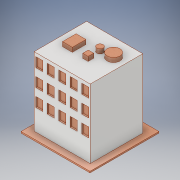
# Autodesk Inventor part: apartment_1
Saved by Autodesk Inventor 2019 (Build 230136000, 136)
## iProperties
Created: 2020-04-29
Part Number: apartment_1
Material: Wood (Oak)
Document SubType Name: Modeling
Designer: infinity
Density: 0.76 g/cm^3
Appearance: White Oak - Natural Medium Gloss
Author: infinity
Autodesk Inventor part; units mm, degrees
ref_plane "YZ Plane" through (0, 0, 0) normal (1, 0, 0) x (0, 1, 0)
ref_plane "XZ Plane" through (0, 0, 0) normal (0, 1, 0) x (-1, 0, 0)
ref_plane "XY Plane" through (0, 0, 0) normal (0, 0, 1) x (1, 0, 0)
sketch "Sketch1" plane through (0, 0, 0) normal (0, 1, 0) x (-1, 0, 0)
  line L0 (0, 0) -> (1219.2, 0)
  line L1 (1219.2, 0) -> (1219.2, -1219.2)
  line L2 (1219.2, -1219.2) -> (0, -1219.2)
  line L3 (0, -1219.2) -> (0, 0)
  dimension "d0" = 1219.2
  dimension "d1" = 1219.2
  constraints: 8 end point, 2 parallel, 1 horizontal, 1 perpendicular
  measures "d0" distance of L0.end L1.end
  measures "d1" distance of L1.end L2.end
extrude "Extrusion1" add sketch "Sketch1" along normal blind 25.4
sketch "Sketch2" plane through (0, 25.4, 0) normal (0, 1, 0) x (1, 0, 0)
  line L0 (-1107.5056, 119.0242) -> (-114.6697, 119.0242)
  line L1 (-114.6697, 119.0242) -> (-114.6697, 1047.9936)
  line L2 (-114.6697, 1047.9936) -> (-1107.5056, 1047.9936)
  line L3 (-1107.5056, 1047.9936) -> (-1107.5056, 119.0242)
  point P0 (0, 0)
  constraints: 8 end point, 2 parallel, 1 horizontal, 1 perpendicular
extrude "Extrusion2" add sketch "Sketch2" along normal blind 1219.2
sketch "Sketch3" plane through (0, 1244.6, 0) normal (0, 1, 0) x (1, 0, 0)
  line L0 (-933.3238, 447.0665) -> (-759.1421, 447.0665)
  line L1 (-759.1421, 447.0665) -> (-759.1421, 688.0179)
  line L2 (-759.1421, 688.0179) -> (-933.3238, 688.0179)
  line L3 (-933.3238, 688.0179) -> (-933.3238, 447.0665)
  line L4 (-576.2513, 447.0665) -> (-480.4513, 447.0665)
  line L5 (-480.4513, 447.0665) -> (-480.4513, 545.7695)
  line L6 (-480.4513, 545.7695) -> (-576.2513, 545.7695)
  line L7 (-576.2513, 545.7695) -> (-576.2513, 447.0665)
  circle A0 centre (-528.3513, 705.4361) radius 55.5572
  circle A1 centre (-317.8817, 734.4664) radius 113.2181
  point P0 (0, 0)
  constraints: 16 end point, 4 parallel, 2 centre point, 2 horizontal, 2 perpendicular, 1 point on line
extrude "Extrusion3" add sketch "Sketch3" along normal blind 76.2
sketch "Sketch4" plane through (-1107.5056, 25.4, -119.0242) normal (0, 0, 1) x (1, 0, 0)
  line L0 (30.4818, 1157.5843) -> (152.4572, 1157.5843)
  line L1 (152.4572, 1157.5843) -> (152.4572, 989.2087)
  line L2 (152.4572, 989.2087) -> (30.4818, 989.2087)
  line L3 (30.4818, 989.2087) -> (30.4818, 1157.5843)
  line L4 (0, 1219.2) -> (992.8359, 1219.2) projected
  line L5 (0, 0) -> (0, 1219.2) projected
  line L6 (233.6818, 1157.5843) -> (355.6572, 1157.5843)
  line L7 (355.6572, 1157.5843) -> (355.6572, 989.2087)
  line L8 (355.6572, 989.2087) -> (233.6818, 989.2087)
  line L9 (233.6818, 989.2087) -> (233.6818, 1157.5843)
  line L10 (436.8818, 1157.5843) -> (558.8572, 1157.5843)
  line L11 (558.8572, 1157.5843) -> (558.8572, 989.2087)
  line L12 (558.8572, 989.2087) -> (436.8818, 989.2087)
  line L13 (436.8818, 989.2087) -> (436.8818, 1157.5843)
  line L14 (640.0818, 1157.5843) -> (762.0572, 1157.5843)
  line L15 (762.0572, 1157.5843) -> (762.0572, 989.2087)
  line L16 (762.0572, 989.2087) -> (640.0818, 989.2087)
  line L17 (640.0818, 989.2087) -> (640.0818, 1157.5843)
  line L18 (843.2818, 1157.5843) -> (965.2572, 1157.5843)
  line L19 (965.2572, 1157.5843) -> (965.2572, 989.2087)
  line L20 (965.2572, 989.2087) -> (843.2818, 989.2087)
  line L21 (843.2818, 989.2087) -> (843.2818, 1157.5843)
  line L22 (30.4818, 852.7843) -> (152.4572, 852.7843)
  line L23 (152.4572, 852.7843) -> (152.4572, 684.4087)
  line L24 (152.4572, 684.4087) -> (30.4818, 684.4087)
  line L25 (30.4818, 684.4087) -> (30.4818, 852.7843)
  line L26 (233.6818, 852.7843) -> (355.6572, 852.7843)
  line L27 (355.6572, 852.7843) -> (355.6572, 684.4087)
  line L28 (355.6572, 684.4087) -> (233.6818, 684.4087)
  line L29 (233.6818, 684.4087) -> (233.6818, 852.7843)
  line L30 (436.8818, 852.7843) -> (558.8572, 852.7843)
  line L31 (558.8572, 852.7843) -> (558.8572, 684.4087)
  line L32 (558.8572, 684.4087) -> (436.8818, 684.4087)
  line L33 (436.8818, 684.4087) -> (436.8818, 852.7843)
  line L34 (640.0818, 852.7843) -> (762.0572, 852.7843)
  line L35 (762.0572, 852.7843) -> (762.0572, 684.4087)
  line L36 (762.0572, 684.4087) -> (640.0818, 684.4087)
  line L37 (640.0818, 684.4087) -> (640.0818, 852.7843)
  line L38 (843.2818, 852.7843) -> (965.2572, 852.7843)
  line L39 (965.2572, 852.7843) -> (965.2572, 684.4087)
  line L40 (965.2572, 684.4087) -> (843.2818, 684.4087)
  line L41 (843.2818, 684.4087) -> (843.2818, 852.7843)
  line L42 (30.4818, 547.9843) -> (152.4572, 547.9843)
  line L43 (152.4572, 547.9843) -> (152.4572, 379.6087)
  line L44 (152.4572, 379.6087) -> (30.4818, 379.6087)
  line L45 (30.4818, 379.6087) -> (30.4818, 547.9843)
  line L46 (233.6818, 547.9843) -> (355.6572, 547.9843)
  line L47 (355.6572, 547.9843) -> (355.6572, 379.6087)
  line L48 (355.6572, 379.6087) -> (233.6818, 379.6087)
  line L49 (233.6818, 379.6087) -> (233.6818, 547.9843)
  line L50 (436.8818, 547.9843) -> (558.8572, 547.9843)
  line L51 (558.8572, 547.9843) -> (558.8572, 379.6087)
  line L52 (558.8572, 379.6087) -> (436.8818, 379.6087)
  line L53 (436.8818, 379.6087) -> (436.8818, 547.9843)
  line L54 (640.0818, 547.9843) -> (762.0572, 547.9843)
  line L55 (762.0572, 547.9843) -> (762.0572, 379.6087)
  line L56 (762.0572, 379.6087) -> (640.0818, 379.6087)
  line L57 (640.0818, 379.6087) -> (640.0818, 547.9843)
  line L58 (843.2818, 547.9843) -> (965.2572, 547.9843)
  line L59 (965.2572, 547.9843) -> (965.2572, 379.6087)
  line L60 (965.2572, 379.6087) -> (843.2818, 379.6087)
  line L61 (843.2818, 379.6087) -> (843.2818, 547.9843)
  point P0 (1107.5056, -25.4)
  dimension "d10" = 203.2
  dimension "d13" = 304.8
  constraints: 120 end point, 2 horizontal, 2 parallel, 1 perpendicular, 1 vertical, 112 other
  measures "d10" distance of L0.start L6.start
  measures "d13" distance of L0.start L22.start
extrude "Extrusion4" cut sketch "Sketch4" against normal blind 25.4
sketch "Sketch5" plane through (-1107.5056, 25.4, -1047.9936) normal (-1, 0, 0) x (0, 0, 1)
  line L0 (81.2848, 304.8) -> (865.1027, 304.8)
  line L1 (865.1027, 304.8) -> (865.1027, 0)
  line L2 (865.1027, 0) -> (81.2848, 0)
  line L3 (81.2848, 0) -> (81.2848, 304.8)
  line L4 (-171.2064, 0) -> (1047.9936, 0) projected
  point P0 (1047.9936, -25.4)
  dimension "d18" = 0
  dimension "d19" = 304.8
  constraints: 8 end point, 2 parallel, 1 horizontal, 1 perpendicular
  measures "d18" distance between parallel lines of L4 L2
  measures "d19" distance between parallel lines of L2 L0
extrude "Extrusion5" cut sketch "Sketch5" against normal blind 609.6
equation "\"d1\" = d0"
body "Solid1"
